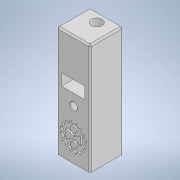
# Autodesk Inventor part: Idle Bearing Mount
Saved by Autodesk Inventor 2022 (Build 260153000, 153)
## iProperties
Created: 2022-04-23
Part Number: Idle Bearing Mount
Material: Generic
Document SubType Name: Modeling
Designer: Nick
Density: 1 g/cm^3
Appearance: Default
Author: Nick
Autodesk Inventor part; units mm, degrees
ref_plane "YZ Plane" through (0, 0, 0) normal (1, 0, 0) x (0, 1, 0)
ref_plane "XZ Plane" through (0, 0, 0) normal (0, 1, 0) x (-1, 0, 0)
ref_plane "XY Plane" through (0, 0, 0) normal (0, 0, 1) x (1, 0, 0)
sketch "Sketch1" plane through (0, 0, 0) normal (0, 0, 1) x (1, 0, 0)
  line L0 (0, 66.05) -> (20, 66.05)
  line L1 (20, 66.05) -> (20, 0)
  line L2 (20, 0) -> (0, 0)
  line L3 (0, 0) -> (0, 66.05)
  line L4 (3, 43.5) -> (17, 43.5)
  line L5 (17, 43.5) -> (17, 36.5)
  line L6 (17, 36.5) -> (3, 36.5)
  line L7 (3, 36.5) -> (3, 43.5)
  point P0 (10, 43.5)
  point P1 (10, 66.05)
  dimension "d1" = 20
  dimension "d2" = 14
  dimension "d3" = 7
  dimension "d4" = 22.55
  dimension "d66" = 36.5
  constraints: 16 end point, 4 parallel, 2 horizontal, 2 midpoint, 2 perpendicular, 1 coincident, 1 vertical alignment
  measures "d1" distance of L1.end L2.end
  measures "d2" distance of L4.start L4.end
  measures "d3" distance of L4.end L5.end
  measures "d4" distance between parallel lines of L4 L0
  measures "d66" distance between parallel lines of L2 L6
extrude "Extrusion1" add sketch "Sketch1" along normal blind 20
sketch "Sketch2" plane through (0, 0, 0) normal (0, -1, 0) x (1, 0, 0)
  line L0 (0, 0) -> (20, 0) projected
  line L1 (20, 0) -> (20, 20) projected
  line L2 (0, 0) -> (0, 20) projected
  line L3 (0, 20) -> (20, 20) projected
  point P0 (10, 4)
  point P1 (16, 16)
  point P2 (4, 16)
  point P3 (10, 0)
  dimension "d9" = 4
  dimension "d12" = 4
  dimension "d13" = 4
  dimension "d14" = 4
  constraints: 1 horizontal alignment, 1 midpoint, 1 vertical alignment
  measures "d9" distance from line of L0 point (10, 4)
  measures "d12" distance from line of L1 point (16, 16)
  measures "d13" distance from line of L3 point (16, 16)
  measures "d14" distance from line of L2 point (4, 16)
hole "Hole1" at (10, 0, 4) at (16, 0, 16) at (4, 0, 16) direction (0, 1, 0) diameter 4 depth 7
sketch "Sketch3" plane through (0, 0, 20) normal (0, 0, 1) x (1, 0, 0)
  line L0 (17, 36.5) -> (3, 36.5) projected
  point P0 (0, 0)
  point P1 (10, 29.5)
  point P2 (10, 36.5)
  dimension "d22" = 7
  constraints: 1 midpoint, 1 vertical alignment
  measures "d22" distance from line of L0 point (10, 29.5)
hole "Hole2" at (10, 29.5, 20) direction (0, 0, -1) diameter 4 depth 8
chamfer "Chamfer1" distance 0.5 angle 45 1 edges at (10, 31.5, 20)
sketch "Sketch4" plane through (0, 66.05, 0) normal (0, 1, 0) x (1, 0, 0)
  line L0 (8, -12) -> (12, -12) projected
  line L1 (12, -19.5) -> (8, -19.5) projected
  line L2 (20, 0) -> (0, 0) projected
  point P0 (10, -6)
  point P1 (10, 0)
  dimension "d33" = 6
  dimension "d34" = 6
  constraints: 1 midpoint, 1 vertical alignment
  measures "d33" distance from line of L0 point (10, -6)
  measures "d34" distance from line of L2 point (10, -6)
hole "Hole3" at (10, 66.05, 6) direction (0, -1, 0) diameter 3.4 depth 40 counterbore diameter 6.5 counterbore depth 20 clearance for "Socket Head Cap Screw" size "M3" standard "Ansi Metric M Profile"
sketch "Sketch5" plane through (3, 36.5, 0) normal (0, 1, 0) x (1, 0, 0)
  circle A0 centre (7, -6) radius 1.7
  circle A1 centre (7, -6) radius 2.5
  circle A2 centre (7, -6) radius 1.7 projected
  point P0 (-3, 0)
  dimension "d42" = 5
  dimension "d67" = 3.4
  constraints: 2 centre point, 2 coincident
  measures "d42" diameter of A1
  measures "d67" diameter of A0
extrude "Extrusion2" add sketch "Sketch5" along normal blind 0.95
chamfer "Chamfer2" distance 0.95 angle 45 1 edges at (7.5, 36.5, 6)
sketch "Sketch6" plane through (3, 43.5, 0) normal (0, -1, 0) x (1, 0, 0)
  circle A0 centre (7, 6) radius 1.7 projected
  circle A1 centre (7, 6) radius 2.5
  point P0 (-3, 0)
  dimension "d48" = 5
  constraints: 1 centre point, 1 coincident
  measures "d48" diameter of A1
extrude "Extrusion3" add sketch "Sketch6" along normal blind 0.95
chamfer "Chamfer3" distance 0.95 angle 45 1 edges at (7.5, 43.5, 6)
sketch "Sketch7" plane through (0, 0, 0) normal (0, -1, 0) x (1, 0, 0)
  circle A0 centre (16, 16) radius 2 projected
  circle A1 centre (10, 4) radius 2 projected
  circle A2 centre (4, 16) radius 2 projected
  line L0 (0, 0) -> (20, 0) projected
  line L1 (20, 0) -> (20, 20) projected
  line L2 (0, 20) -> (20, 20) projected
  line L3 (0, 0) -> (0, 20) projected
  line L4 (15, 17.7321) -> (16, 18.3094)
  line L5 (16, 18.3094) -> (17, 17.7321)
  line L6 (3, 17.7321) -> (4, 18.3094)
  line L7 (4, 18.3094) -> (5, 17.7321)
  line L8 (9, 5.7321) -> (10, 6.3094)
  line L9 (10, 6.3094) -> (11, 5.7321)
  circle A3 centre (10, 4) radius 2 projected
  circle A4 centre (10, 4) radius 2 construction
  line L10 (10, 6.3094) -> (10, 4) construction
  circle A5 centre (16, 16) radius 2 construction
  line L11 (16, 18.3094) -> (16, 16) construction
  line L12 (4, 18.3094) -> (4, 16) construction
  dimension "d54" = 120
  dimension "d55" = 120
  dimension "d56" = 120
  constraints: 18 end point, 4 point on circle, 4 tangent, 3 vertical, 6 other
  measures "d54" angle of L8 L9
  measures "d55" angle of L5 L4
  measures "d56" angle of L7 L6
extrude "Extrusion4" cut sketch "Sketch7" against normal up to surface (7 mm away) contours A0 L4 L5 | A1 L8 L9 | A2 L6 L7
ref_plane "Work Plane2" through (3, 33.5, 0) normal (0, 1, 0) x (1, 0, 0)
sketch "Sketch8" plane through (3, 33.5, 0) normal (0, 1, 0) x (1, 0, 0)
  line L0 (4.25, -4.4123) -> (7, -2.8246)
  line L1 (7, -2.8246) -> (9.75, -4.4123)
  line L2 (9.75, -4.4123) -> (9.75, -7.5877)
  line L3 (9.75, -7.5877) -> (7, -9.1754)
  line L4 (7, -9.1754) -> (4.25, -7.5877)
  line L5 (4.25, -7.5877) -> (4.25, -4.4123)
  line L6 (9.75, -4.4123) -> (9.75, 0.1245)
  line L7 (4.25, -4.4123) -> (4.25, 0)
  line L8 (0, 0) -> (14, 0) projected
  circle A0 centre (7, -6) radius 1.7 projected
  point P0 (-3, 0)
  point P1 (9.75, 0)
  dimension "d60" = 5.5
  constraints: 16 end point, 2 vertical, 1 coincident, 1 point on line, 15 other
  measures "d60" distance between parallel lines of L5 L2
extrude "Extrusion5" cut sketch "Sketch8" against normal blind 2.5 contours L7 L8 L6 L1 L0 | L0 L1 L2 L3 L4 L5 | A0
chamfer "Chamfer4" distance 0.95 angle 45 8 edges at (0, 33.025, 20) (20, 33.025, 20) (10, 66.05, 20) (10, 66.05, 0) (0, 33.025, 0) (20, 33.025, 0) (20, 66.05, 10) (0, 66.05, 10)
sketch "Sketch9" plane through (0, 0, 20) normal (0, 0, 1) x (1, 0, 0)
  arc A0 (5.9151, 20.4046) -> (8.0061, 21.2707) centre (6.9299, 20.9118) ccw
  arc A1 (5.9151, 20.4046) -> (5.1842, 19.9162) centre (10, 13.5) ccw
  arc A2 (3.5838, 18.3158) -> (5.1842, 19.9162) centre (4.3273, 19.1727) ccw
  arc A3 (3.5838, 18.3158) -> (3.0954, 17.5849) centre (10, 13.5) ccw
  arc A4 (2.2293, 15.4939) -> (3.0954, 17.5849) centre (2.5882, 16.5701) ccw
  arc A5 (2.2293, 15.4939) -> (2.0578, 14.6316) centre (10, 13.5) ccw
  arc A6 (2.0578, 12.3684) -> (2.0578, 14.6316) centre (1.9775, 13.5) ccw
  arc A7 (2.0578, 12.3684) -> (2.2293, 11.5061) centre (10, 13.5) ccw
  arc A8 (3.0954, 9.4151) -> (2.2293, 11.5061) centre (2.5882, 10.4299) ccw
  arc A9 (3.0954, 9.4151) -> (3.5838, 8.6842) centre (10, 13.5) ccw
  arc A10 (5.1842, 7.0838) -> (3.5838, 8.6842) centre (4.3273, 7.8273) ccw
  arc A11 (5.1842, 7.0838) -> (5.9151, 6.5954) centre (10, 13.5) ccw
  arc A12 (8.0061, 5.7293) -> (5.9151, 6.5954) centre (6.9299, 6.0882) ccw
  arc A13 (8.0061, 5.7293) -> (8.8684, 5.5578) centre (10, 13.5) ccw
  arc A14 (11.1316, 5.5578) -> (8.8684, 5.5578) centre (10, 5.4775) ccw
  arc A15 (11.1316, 5.5578) -> (11.9939, 5.7293) centre (10, 13.5) ccw
  arc A16 (14.0849, 6.5954) -> (11.9939, 5.7293) centre (13.0701, 6.0882) ccw
  arc A17 (14.0849, 6.5954) -> (14.8158, 7.0838) centre (10, 13.5) ccw
  arc A18 (16.4162, 8.6842) -> (14.8158, 7.0838) centre (15.6727, 7.8273) ccw
  arc A19 (16.4162, 8.6842) -> (16.9046, 9.4151) centre (10, 13.5) ccw
  arc A20 (17.7707, 11.5061) -> (16.9046, 9.4151) centre (17.4118, 10.4299) ccw
  arc A21 (17.7707, 11.5061) -> (17.9422, 12.3684) centre (10, 13.5) ccw
  arc A22 (17.9422, 14.6316) -> (17.9422, 12.3684) centre (18.0225, 13.5) ccw
  arc A23 (17.9422, 14.6316) -> (17.7707, 15.4939) centre (10, 13.5) ccw
  arc A24 (16.9046, 17.5849) -> (17.7707, 15.4939) centre (17.4118, 16.5701) ccw
  arc A25 (16.9046, 17.5849) -> (16.4162, 18.3158) centre (10, 13.5) ccw
  arc A26 (14.8158, 19.9162) -> (16.4162, 18.3158) centre (15.6727, 19.1727) ccw
  arc A27 (14.8158, 19.9162) -> (14.0849, 20.4046) centre (10, 13.5) ccw
  arc A28 (11.9939, 21.2707) -> (14.0849, 20.4046) centre (13.0701, 20.9118) ccw
  arc A29 (11.9939, 21.2707) -> (11.1316, 21.4422) centre (10, 13.5) ccw
  arc A30 (8.8684, 21.4422) -> (11.1316, 21.4422) centre (10, 21.5225) ccw
  arc A31 (8.8684, 21.4422) -> (8.0061, 21.2707) centre (10, 13.5) ccw
  circle A32 centre (10, 9.4589) radius 1.8673
  circle A33 centre (10, 17.5411) radius 1.8673
  arc A34 (10.1862, 12.9107) -> (9.8138, 12.9107) centre (10, 12.5093) ccw
  line L0 (10.1862, 12.9107) -> (13.8757, 11.1989)
  arc A35 (13.8757, 11.1989) -> (14.5044, 11.6003) centre (14.0619, 11.6003) ccw
  line L1 (14.5044, 11.6003) -> (14.5044, 15.3997)
  arc A36 (14.5044, 15.3997) -> (13.8757, 15.8011) centre (14.0619, 15.3997) ccw
  line L2 (13.8757, 15.8011) -> (10.1862, 14.0893)
  arc A37 (9.8138, 14.0893) -> (10.1862, 14.0893) centre (10, 14.4907) ccw
  line L3 (9.8138, 14.0893) -> (6.1243, 15.8011)
  arc A38 (6.1243, 15.8011) -> (5.4956, 15.3997) centre (5.9381, 15.3997) ccw
  line L4 (5.4956, 15.3997) -> (5.4956, 11.6003)
  arc A39 (5.4956, 11.6003) -> (6.1243, 11.1989) centre (5.9381, 11.6003) ccw
  line L5 (6.1243, 11.1989) -> (9.8138, 12.9107)
  line L6 (0.95, 0) -> (19.05, 0) projected
  circle A40 centre (10, 29.5) radius 2.5 projected
  line L7 (6.5965, 27) -> (15.1739, 27) construction
  point P0 (0, 0)
  point P1 (10, 0)
  point P2 (3.5838, 18.3158)
  point P3 (2.2293, 15.4939)
  point P4 (2.0578, 14.6316)
  point P5 (2.0578, 12.3684)
  point P6 (2.2293, 11.5061)
  point P7 (3.0954, 9.4151)
  point P8 (3.5838, 8.6842)
  point P9 (5.1842, 7.0838)
  point P10 (5.9151, 6.5954)
  point P11 (8.0061, 5.7293)
  point P12 (8.8684, 5.5578)
  point P13 (11.1316, 5.5578)
  point P14 (11.9939, 5.7293)
  point P15 (14.8158, 7.0838)
  point P16 (16.9046, 9.4151)
  point P17 (17.7707, 11.5061)
  point P18 (17.9422, 12.3684)
  point P19 (17.9422, 14.6316)
  point P20 (17.7707, 15.4939)
  point P21 (16.9046, 17.5849)
  point P22 (16.4162, 18.3158)
  point P23 (14.0849, 20.4046)
  point P24 (11.9939, 21.2707)
  point P25 (11.1316, 21.4422)
  point P26 (8.8684, 21.4422)
  point P27 (8.0061, 21.2707)
  point P28 (5.9151, 20.4046)
  point P29 (5.1842, 19.9162)
  point P30 (6.1243, 11.1989)
  point P31 (5.4956, 15.3997)
  point P32 (9.8138, 14.0893)
  point P33 (13.8757, 15.8011)
  dimension "d69" = 13.5
  dimension "d70" = 13.5
  constraints: 76 point on circle, 40 centre point, 14 end point, 1 horizontal, 1 midpoint, 1 tangent, 1 vertical alignment
  measures "d69" distance from line of point (10, 13.5) L7
  measures "d70" distance from line of L6 point (10, 13.5)
extrude "Extrusion6" cut sketch "Sketch9" against normal blind 1 contours A0 A31 A30 A29 A28 A27 A26 A25 A24 A23 A22 A21 A20 A19 A18 A17 A16 A15 A14 A13 A12 A11 A10 A9 A8 A7 A6 A5 A4 A3 A2 A1
chamfer "Chamfer5" distance 1.55 angle 45 1 edges at (10, 46.05, 4.3)
equation "\"d9\" = d12"
equation "\"d13\" = d12"
equation "\"d14\" = d12"
equation "\"d33\" = d34"
equation "\"d69\" = d70"
equation "\"MotorHeight\" = MotorHeightBase"
equation "\"MotorHeightBase\" = 28"
body "Solid1"
